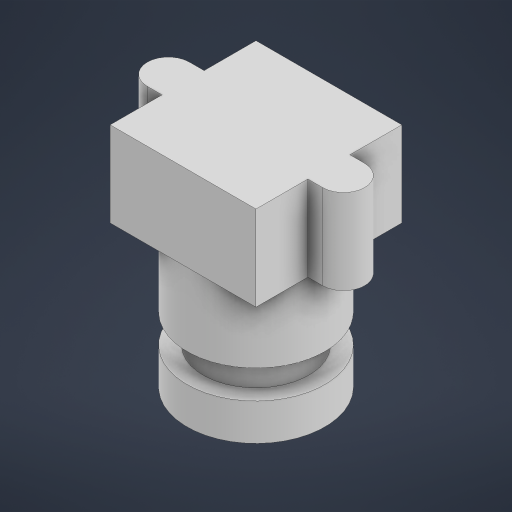
# Autodesk Inventor part: cum
Saved by Autodesk Inventor 2024 (Build 280153000, 153)
## iProperties
Created: 2023-05-15
Part Number: cum
Material: Типовые
Document SubType Name: Modeling
Designer: user
Density: 1 g/cm^3
Appearance: По умолчанию
Author: user
Autodesk Inventor part; units mm, degrees
ref_plane "YZ Plane" through (0, 0, 0) normal (1, 0, 0) x (0, 1, 0)
ref_plane "XZ Plane" through (0, 0, 0) normal (0, 1, 0) x (-1, 0, 0)
ref_plane "XY Plane" through (0, 0, 0) normal (0, 0, 1) x (1, 0, 0)
sketch "Эскиз1" plane through (0, 0, 0) normal (0, 0, 1) x (1, 0, 0)
  line L0 (0, 0) -> (16.3, 0)
  line L1 (16.3, 16.3) -> (0, 16.3)
  line L2 (0, 10.5) -> (-1.65, 10.5)
  line L3 (0, 5.8) -> (-1.65, 5.8)
  line L4 (16.3, 10.5) -> (17.95, 10.5)
  line L5 (16.3, 5.8) -> (17.95, 5.8)
  arc A0 (-1.65, 10.5) -> (-1.65, 5.8) centre (-1.65, 8.15) ccw
  arc A1 (17.95, 5.8) -> (17.95, 10.5) centre (17.95, 8.15) ccw
  line L6 (0, 16.3) -> (0, 10.5)
  line L7 (0, 5.8) -> (0, 0)
  line L8 (16.3, 0) -> (16.3, 5.8)
  line L9 (16.3, 10.5) -> (16.3, 16.3)
  point P0 (-4, 8.15)
  dimension "d0" = 4.7
  dimension "d1" = 4
  dimension "d2" = 16.3
  dimension "d3" = 16.3
  dimension "d4" = 4.7
  constraints: 20 end point, 5 parallel, 5 point on circle, 4 horizontal, 4 perpendicular, 4 tangent, 2 centre point, 2 collinear, 2 vertical alignment, 1 horizontal alignment
  measures "d0" distance of L3.start L2.start
  measures "d1" horizontal distance of L2.start point (-4, 8.15)
  measures "d2" distance of L1.start L1.end
  measures "d3" distance of L0.end L1.start
  measures "d4" distance of L5.start L4.start
extrude "Выдавливание1" add sketch "Эскиз1" against normal blind 9.5
sketch "Эскиз2" plane through (0, 0, -9.5) normal (0, 0, -1) x (-1, 0, 0)
  circle A0 centre (-8.15, 8.15) radius 7.7
  arc A1 (1.65, 5.8) -> (1.65, 10.5) centre (1.65, 8.15) ccw projected
  line L0 (0, 16.3) -> (-16.3, 16.3) projected
  point P0 (0, 0)
  point P1 (4, 8.15)
  point P2 (-8.15, 16.3)
  dimension "d7" = 15.4
  constraints: 1 centre point, 1 horizontal alignment, 1 midpoint, 1 point on circle, 1 vertical alignment
  measures "d7" diameter of A0
extrude "Выдавливание2" add sketch "Эскиз2" along normal blind 8.6
sketch "Эскиз3" plane through (8.15, 8.15, -18.1) normal (0, 0, -1) x (-1, 0, 0)
  circle A0 centre (0, 0) radius 5.9
  dimension "d10" = 11.8
  constraints: 1 centre point
  measures "d10" diameter of A0
extrude "Выдавливание3" add sketch "Эскиз3" along normal blind 3.2
sketch "Эскиз4" plane through (8.15, 8.15, -21.3) normal (0, 0, -1) x (-1, 0, 0)
  circle A0 centre (0, 0) radius 7.7 projected
extrude "Выдавливание4" add sketch "Эскиз4" along normal blind 4.1
equation "\"d4\" = d0"
